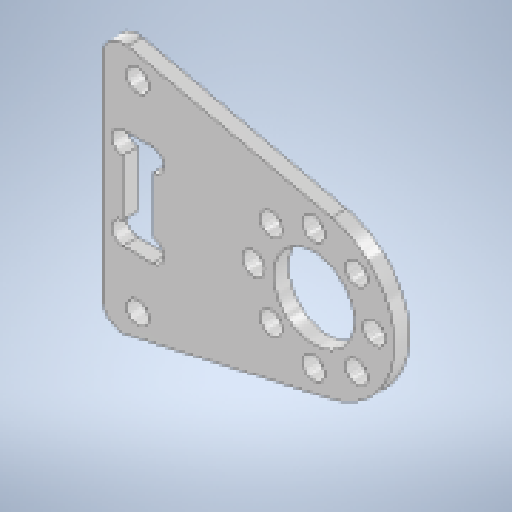
# Autodesk Inventor part: kata_new
Saved by Autodesk Inventor 2024 (Build 280153000, 153)
## iProperties
Created: 2023-12-16
Part Number: kata_new
Material: アルミニウム 2014-T4
Document SubType Name: Modeling
Designer: right
Density: 2.8 g/cm^3
Appearance: サテン
Mass: 1.75294 g
Surface Area: 11.5978 cm^2
Volume: 0.62605 cm^3
Author: right
Autodesk Inventor part; units mm, degrees
ref_plane "YZ Plane" through (0, 0, 0) normal (1, 0, 0) x (0, 1, 0)
ref_plane "XZ Plane" through (0, 0, 0) normal (0, 1, 0) x (-1, 0, 0)
ref_plane "XY Plane" through (0, 0, 0) normal (0, 0, 1) x (1, 0, 0)
sketch "スケッチ1" plane through (0, 0, 0) normal (0, 0, 1) x (1, 0, 0)
  circle A0 centre (8.8, 8.8) radius 8 projected
  circle A1 centre (8.8, 8.8) radius 8 projected
  circle A2 centre (2.8, 8.8) radius 0.825 projected
  circle A3 centre (4.5574, 4.5574) radius 0.825 projected
  circle A4 centre (8.8, 2.8) radius 0.825 projected
  circle A5 centre (13.0426, 4.5574) radius 0.825 projected
  circle A6 centre (14.8, 8.8) radius 0.825 projected
  circle A7 centre (13.0426, 13.0426) radius 0.825 projected
  circle A8 centre (8.8, 14.8) radius 0.825 projected
  circle A9 centre (4.5574, 13.0426) radius 0.825 projected
  circle A10 centre (8.8, 8.8) radius 4 projected
  circle A11 centre (2.8, 8.8) radius 1.1
  circle A12 centre (4.5574, 4.5574) radius 1.1
  circle A13 centre (8.8, 2.8) radius 1.1
  circle A14 centre (13.0426, 4.5574) radius 1.1
  circle A15 centre (14.8, 8.8) radius 1.1
  circle A16 centre (13.0426, 13.0426) radius 1.1
  circle A17 centre (8.8, 14.8) radius 1.1
  circle A18 centre (4.5574, 13.0426) radius 1.1
  line L0 (8.8, 0.8) -> (-2.0211, 0.8)
  line L1 (8.8, 16.8) -> (-2.0211, 16.8)
  line L2 (-10.2, 3.8) -> (-7.2, 3.8)
  line L3 (-7.2, 3.8) -> (-7.2, 13.8)
  line L4 (-7.2, 13.8) -> (-10.2, 13.8)
  line L5 (-10.2, 13.8) -> (-10.2, 3.8)
  line L6 (0.8, 16.8) -> (0.8, 0.8) construction
  circle A19 centre (-10.2, 4.9) radius 1.1
  line L7 (-10.2, 8.8) -> (-7.2, 8.8) construction
  line L8 (-8.7, 8.8) -> (-8.7, 3.8) construction
  circle A20 centre (-7.2, 4.9) radius 1.1
  circle A21 centre (-10.2, 12.7) radius 1.1
  circle A22 centre (-7.2, 12.7) radius 1.1
  circle A23 centre (-8.7, -1.2) radius 1.1
  circle A24 centre (-8.7, 18.8) radius 1.1
  line L9 (-12.2, -4.2) -> (-3.1, -4.2) construction
  line L10 (-3.1, -4.2) -> (-3.1, 21.8)
  line L11 (-3.1, 21.8) -> (-12.2, 21.8) construction
  line L12 (-12.2, 21.8) -> (-12.2, -4.2)
  line L13 (-12.2, -4.2) -> (10.5805, 1.0007)
  line L14 (-12.2, 21.8) -> (10.5805, 16.5993)
  point P0 (0, 0)
  point P1 (-12.2, 8.8)
  point P2 (-7.2, 11.6)
  point P3 (-7.2, 6)
  point P4 (-7.2, 3.8)
  point P5 (-10.2, 6)
  point P6 (-10.2, 11.6)
  point P7 (-10.2, 13.8)
  point P8 (-7.2, 13.8)
  point P9 (-0.1, 16.8)
  point P10 (-3.1, 19.7225)
  point P11 (-3.1, -2.1225)
  dimension "d7" = 2.2
  dimension "d0" = 2.2
  dimension "d3" = 360
  dimension "d5" = 3
  dimension "d6" = 10
  dimension "d8" = 8
  dimension "d9" = 2.2
  dimension "d10" = 5
  dimension "d11" = 3
  dimension "d12" = 2
  dimension "d13" = 3
  constraints: 30 end point, 13 centre point, 7 horizontal, 5 midpoint, 5 symmetric about line, 4 parallel, 3 perpendicular, 3 point on line, 2 horizontal alignment, 2 point on circle, 2 tangent, 2 vertical, 1 coincident, 1 vertical alignment, 27 other
  measures "d0" diameter of A11
  measures "d5" distance of L4.end L3.end
  measures "d6" distance of L3.end L2.end
  measures "d8" distance from line of L6 A22.centre
  measures "d9" diameter of A23
  measures "d10" distance of L8.end A23.centre
  measures "d11" distance edge to line of A22 L10
  measures "d12" distance from line of L12 A21.centre
  measures "d13" distance from line of L11 A24.centre
extrude "押し出し1" add sketch "スケッチ1" along normal blind 1.5 contours A0 | A0 L13 L10 L14 | L10 L13 L12 L14
fillet "フィレット1" radius 2 2 edges at (-12.2, 21.8, 0.75) (-12.2, -4.2, 0.75)
